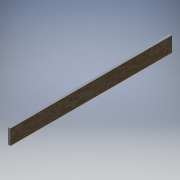
# Autodesk Inventor part: Euph wheel mount front
Saved by Autodesk Inventor 2018.2 (Build 222227000, 227)
## iProperties
Created: 2018-02-27
Part Number: Euph wheel mount front
Material: Generic
Document SubType Name: Modeling
Designer: owner
Density: 1 g/cm^3
Appearance: Default
Author: owner
Autodesk Inventor part; units mm, degrees
ref_plane "YZ Plane" through (0, 0, 0) normal (1, 0, 0) x (0, 1, 0)
ref_plane "XZ Plane" through (0, 0, 0) normal (0, 1, 0) x (-1, 0, 0)
ref_plane "XY Plane" through (0, 0, 0) normal (0, 0, 1) x (1, 0, 0)
sketch "Sketch1" plane through (0, 0, 0) normal (1, 0, 0) x (0, 1, 0)
  line L0 (378.3449, 1023.826) -> (378.3449, 1049.226) projected
  line L1 (251.3449, 1049.226) -> (378.3449, 1049.226) projected
  line L2 (251.3449, 1023.826) -> (251.3449, 1049.226) projected
  line L3 (251.3449, 947.626) -> (270.3949, 947.626) projected
  line L4 (251.3449, 1023.826) -> (270.3949, 1023.826) projected
  line L5 (251.3449, 947.626) -> (251.3449, 1023.826) projected
  line L6 (378.3449, 1049.226) -> (378.3449, -308.7342) projected
  line L7 (397.3949, -308.7342) -> (378.3449, -308.7342) projected
  line L8 (397.3949, 1049.226) -> (397.3949, -308.7342) projected
  line L9 (251.3449, -308.7342) -> (378.3449, -308.7342) projected
  line L10 (378.3449, -308.7342) -> (378.3449, -283.3342) projected
  line L11 (251.3449, -308.7342) -> (251.3449, -283.3342) projected
  line L12 (251.3449, -283.3342) -> (251.3449, -207.1342) projected
  line L13 (378.3449, 1049.226) -> (251.3449, 1049.226)
  line L14 (251.3449, 1049.226) -> (251.3449, -308.7342)
  line L15 (251.3449, -308.7342) -> (378.3449, -308.7342)
  line L16 (378.3449, -308.7342) -> (378.3449, 1049.226)
  point P0 (0, 0)
  point P1 (270.3949, -283.3342)
  point P2 (270.3949, -207.1342)
  constraints: 8 end point, 2 parallel, 1 horizontal, 1 perpendicular
extrude "Extrusion1" add sketch "Sketch1" along normal blind 19.05
body "Solid1"
